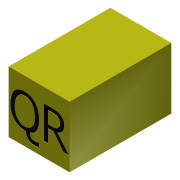
# Autodesk Inventor part: Container 1 1 2 and half
Saved by Autodesk Inventor 2015 (Build 190159000, 159)
## iProperties
Created: 2015-03-07
Part Number: Container 1 1 2 and half
Material: Generic
Document SubType Name: Modeling
Designer: Vukica
Density: 1 g/cm^3
Appearance: Yellow
Author: Vukica
Autodesk Inventor part; units mm, degrees
ref_plane "YZ Plane" through (0, 0, 0) normal (1, 0, 0) x (0, 1, 0)
ref_plane "XZ Plane" through (0, 0, 0) normal (0, 1, 0) x (-1, 0, 0)
ref_plane "XY Plane" through (0, 0, 0) normal (0, 0, 1) x (1, 0, 0)
sketch "Sketch1" plane through (0, 0, 0) normal (0, 0, 1) x (1, 0, 0)
  line L0 (0, 0) -> (38.1, 0)
  line L1 (38.1, 0) -> (38.1, 38.1)
  line L2 (38.1, 38.1) -> (0, 38.1)
  line L3 (0, 38.1) -> (0, 0)
  dimension "d0" = 38.1
  dimension "d1" = 38.1
  constraints: 8 end point, 2 parallel, 1 horizontal, 1 perpendicular
  measures "d0" distance of L1.end L2.end
  measures "d1" distance of L2.end L0.start
extrude "Extrusion1" add sketch "Sketch1" along normal blind 63.5
sketch "Sketch2" plane through (0, 0, 63.5) normal (0, 0, 1) x (1, 0, 0)
  line L0 (0.1215, 29.4926) -> (23.3191, 29.4926) construction
  line L1 (23.3191, 29.4926) -> (23.3191, 13.1802) construction
  line L2 (23.3191, 13.1802) -> (0.1215, 13.1802) construction
  line L3 (0.1215, 13.1802) -> (0.1215, 29.4926) construction
  spline S0 degree 2 poles (19.0583, 3.7715) (18.3173, 3.5904) (16.7036, 3.3928) (15.8967, 3.3928) knots 0 0 0 1 2 2 2
  spline S1 degree 2 poles (15.8967, 3.3928) (13.6078, 3.3928) (10.7591, 5.9451) (10.6273, 8.3164) knots 0 0 0 1 2 2 2
  spline S2 degree 2 poles (10.6273, 8.3164) (10.4462, 8.3164) (10.1333, 8.3164) (10.0016, 8.3164) knots 0 0 0 1 2 2 2
  spline S3 degree 2 poles (10.0016, 8.3164) (7.9432, 8.3164) (4.6334, 9.716) (3.4478, 11.0828) knots 0 0 0 1 2 2 2
  spline S4 degree 2 poles (3.4478, 11.0828) (2.2787, 12.4331) (1.0272, 16.3851) (1.0272, 18.888) knots 0 0 0 1 2 2 2
  spline S5 degree 2 poles (1.0272, 18.888) (1.0272, 21.4569) (2.2951, 25.343) (3.4643, 26.7262) knots 0 0 0 1 2 2 2
  spline S6 degree 2 poles (3.4643, 26.7262) (4.6499, 28.093) (7.9597, 29.4926) (10.0016, 29.4926) knots 0 0 0 1 2 2 2
  spline S7 degree 2 poles (10.0016, 29.4926) (12.0764, 29.4926) (15.4027, 28.0436) (16.5554, 26.7262) knots 0 0 0 1 2 2 2
  spline S8 degree 2 poles (16.5554, 26.7262) (17.708, 25.3924) (18.9924, 21.4239) (18.9924, 18.888) knots 0 0 0 1 2 2 2
  spline S9 degree 2 poles (18.9924, 18.888) (18.9924, 14.936) (15.9132, 9.7984) (13.2291, 8.8927) knots 0 0 0 1 2 2 2
  spline S10 degree 2 poles (13.2291, 8.8927) (13.2949, 8.1352) (13.6901, 6.9167) (14.003, 6.5709) knots 0 0 0 1 2 2 2
  spline S11 degree 2 poles (14.003, 6.5709) (14.3817, 6.1427) (15.4191, 5.7475) (16.3413, 5.7475) knots 0 0 0 1 2 2 2
  spline S12 degree 2 poles (16.3413, 5.7475) (16.8847, 5.7475) (18.3667, 6.0933) (18.696, 6.2251) knots 0 0 0 1 2 2 2
  line L4 (18.696, 6.2251) -> (19.0583, 6.2251)
  line L5 (19.0583, 6.2251) -> (19.0583, 3.7715)
  spline S13 degree 2 poles (16.1766, 18.888) (16.1766, 20.9134) (15.3039, 24.0257) (14.5135, 25.0466) knots 0 0 0 1 2 2 2
  spline S14 degree 2 poles (14.5135, 25.0466) (13.7066, 26.1005) (11.4342, 27.1544) (10.018, 27.1544) knots 0 0 0 1 2 2 2
  spline S15 degree 2 poles (10.018, 27.1544) (8.5525, 27.1544) (6.346, 26.1334) (5.5062, 25.0466) knots 0 0 0 1 2 2 2
  spline S16 degree 2 poles (5.5062, 25.0466) (4.6993, 24.0092) (3.843, 20.864) (3.843, 18.888) knots 0 0 0 1 2 2 2
  spline S17 degree 2 poles (3.843, 18.888) (3.843, 14.8866) (7.2022, 10.6217) (10.018, 10.6217) knots 0 0 0 1 2 2 2
  spline S18 degree 2 poles (10.018, 10.6217) (12.8339, 10.6217) (16.1766, 14.8866) (16.1766, 18.888) knots 0 0 0 1 2 2 2
  line L6 (37.6822, 8.7445) -> (34.1748, 8.7445)
  line L7 (34.1748, 8.7445) -> (27.7528, 16.8297)
  line L8 (27.7528, 16.8297) -> (24.657, 16.8297)
  line L9 (24.657, 16.8297) -> (24.657, 8.7445)
  line L10 (24.657, 8.7445) -> (21.9565, 8.7445)
  line L11 (21.9565, 8.7445) -> (21.9565, 29.0645)
  line L12 (21.9565, 29.0645) -> (27.1929, 29.0645)
  spline S19 degree 2 poles (27.1929, 29.0645) (28.9384, 29.0645) (31.2931, 28.6858) (32.3635, 27.9942) knots 0 0 0 1 2 2 2
  spline S20 degree 2 poles (32.3635, 27.9942) (33.4338, 27.3026) (34.6688, 25.1454) (34.6688, 23.5481) knots 0 0 0 1 2 2 2
  spline S21 degree 2 poles (34.6688, 23.5481) (34.6688, 21.3251) (32.3964, 18.3117) (30.4533, 17.5872) knots 0 0 0 1 2 2 2
  line L13 (30.4533, 17.5872) -> (37.6822, 8.7445)
  spline S22 degree 2 poles (31.853, 23.3341) (31.853, 24.2233) (31.2273, 25.59) (30.5686, 26.0346) knots 0 0 0 1 2 2 2
  spline S23 degree 2 poles (30.5686, 26.0346) (29.9922, 26.4133) (28.4608, 26.7262) (27.3411, 26.7262) knots 0 0 0 1 2 2 2
  line L14 (27.3411, 26.7262) -> (24.657, 26.7262)
  line L15 (24.657, 26.7262) -> (24.657, 19.0856)
  line L16 (24.657, 19.0856) -> (27.0282, 19.0856)
  spline S24 degree 2 poles (27.0282, 19.0856) (28.1974, 19.0856) (30.0581, 19.4973) (30.7003, 20.1395) knots 0 0 0 1 2 2 2
  spline S25 degree 2 poles (30.7003, 20.1395) (31.2931, 20.6994) (31.853, 22.2802) (31.853, 23.3341) knots 0 0 0 1 2 2 2
  point P0 (0, 0)
  constraints: 2 other
extrude "Extrusion2" cut sketch "Sketch2" against normal blind 0.254
equation "\"d1\" = d0"
body "Solid1"
